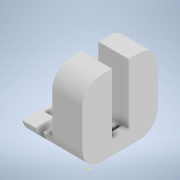
# Autodesk Inventor part: Intsragam
Saved by Autodesk Inventor 2020 (Build 240168000, 168)
## iProperties
Created: 2020-01-07
Part Number: Intsragam
Material: Générique
Document SubType Name: Modeling
Designer: laura
Density: 1 g/cm^3
Appearance: Par défaut
Author: laura
Autodesk Inventor part; units mm, degrees
ref_plane "YZ Plane" through (0, 0, 0) normal (1, 0, 0) x (0, 1, 0)
ref_plane "XZ Plane" through (0, 0, 0) normal (0, 1, 0) x (-1, 0, 0)
ref_plane "XY Plane" through (0, 0, 0) normal (0, 0, 1) x (1, 0, 0)
sketch "Esquisse1" plane through (0, 0, 0) normal (0, 1, 0) x (-1, 0, 0)
  line L0 (0, 0) -> (-40, 0)
  line L1 (-40, 0) -> (-40, -80)
  line L2 (-40, -80) -> (0, -80)
  line L3 (0, -80) -> (0, 0)
  dimension "d0" = 80
  dimension "d4" = 40
  constraints: 8 end point, 2 parallel, 1 horizontal, 1 perpendicular
  measures "d0" distance between parallel lines of L2 L0
  measures "d4" distance between parallel lines of L1 L3
extrude "Extrusion1" add sketch "Esquisse1" along normal blind 80
sketch "Esquisse2" plane through (40, 0, 0) normal (1, 0, 0) x (0, 0, -1)
  point P0 (0, 0)
sketch "Esquisse3" plane through (40, 0, 0) normal (1, 0, 0) x (0, 0, -1)
  line L0 (0, 80) -> (80, 80) projected
  line L1 (20, 20) -> (60, 20)
  line L2 (60, 20) -> (60, 80)
  line L3 (60, 80) -> (20, 80)
  line L4 (20, 80) -> (20, 20)
  line L5 (0, 0) -> (80, 0) projected
  line L6 (80, 0) -> (80, 80) projected
  line L7 (0, 0) -> (0, 80) projected
  point P0 (20, 80)
  dimension "d9" = 20
  dimension "d10" = 20
  dimension "d11" = 20
  constraints: 8 end point, 2 parallel, 1 horizontal, 1 perpendicular, 1 point on line
  measures "d9" distance between parallel lines of L5 L1
  measures "d10" distance between parallel lines of L6 L2
  measures "d11" distance between parallel lines of L7 L4
extrude "Extrusion2" cut sketch "Esquisse3" against normal blind 80 contours L0 L2 L1 L4
sketch "Esquisse4" plane through (40, 20, -20) normal (0, 1, 0) x (1, 0, 0)
  line L0 (0, 40) -> (-40, 40) projected
  line L1 (0, 0) -> (-5, 0)
  line L2 (-5, 40) -> (0, 40)
  line L3 (0, 40) -> (0, 0)
  line L4 (-5, 40) -> (-10, 40)
  line L5 (-9, 10) -> (-12, 10)
  line L6 (-12, 10) -> (-12, 30)
  line L7 (-12, 30) -> (-9, 30)
  line L8 (-9, 10) -> (-9, 30)
  point P0 (-40, -20)
  dimension "d19" = 20
  dimension "d21" = 9
  dimension "d22" = 3
  constraints: 16 end point, 2 horizontal, 2 vertical, 1 parallel, 1 point on line
  measures "d19" distance of L5.end L6.end
  measures "d21" distance between parallel lines of L8 L3
  measures "d22" distance of L5.start L5.end
extrude "Extrusion3" cut sketch "Esquisse4" against normal blind 10
sketch "Esquisse6" plane through (40, 20, -20) normal (0, 0, -1) x (-1, 0, 0)
  line L0 (40, 60) -> (40, 0) projected
  line L1 (0, 60) -> (40, 60) projected
  line L2 (0, 0) -> (0, 60) projected
  line L3 (0, 0) -> (40, 0) projected
  point P0 (40, -20)
extrude "Extrusion4" add sketch "Esquisse6" along normal blind 9
sketch "Esquisse7" plane through (40, 20, -60) normal (0, 0, 1) x (1, 0, 0)
  line L0 (-40, 0) -> (-40, 60) projected
  line L1 (0, 0) -> (-40, 0) projected
  line L2 (0, 60) -> (0, 0) projected
  line L3 (-40, 60) -> (0, 60) projected
  point P0 (-40, -20)
extrude "Extrusion5" add sketch "Esquisse7" along normal blind 9
sketch "Esquisse8" plane through (0, 80, 0) normal (0, 1, 0) x (1, 0, 0)
  line L0 (40, 51) -> (40, 80) projected
  line L1 (40, 80) -> (0, 80) projected
  line L2 (0, 80) -> (0, 51) projected
  line L3 (40, 51) -> (0, 51) projected
  point P0 (0, 0)
extrude "Extrusion6" add sketch "Esquisse8" along normal blind 20
sketch "Esquisse9" plane through (0, 80, 0) normal (0, 1, 0) x (1, 0, 0)
  line L0 (0, 29) -> (0, 0) projected
  line L1 (0, 0) -> (40, 0) projected
  line L2 (40, 0) -> (40, 29) projected
  line L3 (0, 29) -> (40, 29) projected
extrude "Extrusion7" add sketch "Esquisse9" along normal blind 20
sketch "Esquisse10" plane through (0, 0, 0) normal (0, 0, 1) x (1, 0, 0)
  line L0 (0, 0) -> (40, 0) projected
  line L1 (40, 0) -> (40, 100) projected
  line L2 (0, 100) -> (40, 100) projected
  line L3 (0, 0) -> (0, 100) projected
extrude "Extrusion8" add sketch "Esquisse10" along normal blind 10
sketch "Esquisse11" plane through (40, 0, -80) normal (0, 0, -1) x (-1, 0, 0)
  line L0 (0, 0) -> (40, 0) projected
  line L1 (40, 0) -> (40, 100) projected
  line L2 (0, 100) -> (40, 100) projected
  line L3 (0, 0) -> (0, 100) projected
extrude "Extrusion9" add sketch "Esquisse11" along normal blind 10
sketch "Esquisse12" plane through (0, 20, -51) normal (-1, 0, 0) x (0, 0, 1)
  line L0 (22, 80) -> (61, 80) projected
  line L1 (61, 80) -> (36, 80)
  line L2 (61, 80) -> (61, 55)
  line L3 (61, 80) -> (61, -20) projected
  arc A0 (61, 55) -> (36, 80) centre (36, 55) ccw
  point P0 (51, -20)
  dimension "d35" = 25
  dimension "d36" = 25
  constraints: 4 end point, 2 point on circle, 2 point on line, 1 centre point, 1 tangent
  measures "d35" distance of L0.end L1.end
  measures "d36" distance of L0.end L2.end
ref_plane "Plan de construction1" through (40, 0, -40) normal (0, 0, -1) x (-1, 0, 0)
extrude "Extrusion10" cut sketch "Esquisse12" against normal up to surface (40 mm away)
mirror "Symétrie1" about plane through (40, 0, -40) normal (0, 0, -1) of "Extrusion10"
ref_plane "Plan de construction2" through (0, 50, 0) normal (0, 1, 0) x (1, 0, 0)
mirror "Symétrie2" about plane through (0, 50, 0) normal (0, 1, 0) of "Extrusion10", "Symétrie1"
sketch "Esquisse13" plane through (0, 20, -51) normal (-1, 0, 0) x (0, 0, 1)
  line L0 (11, -10) -> (-14, -10)
  line L1 (11, -10) -> (36, -10)
  line L2 (-14, -10) -> (-14, 0)
  line L3 (-14, 0) -> (-38.4949, 0)
  line L4 (36, -10) -> (36, 0)
  line L5 (36, 0) -> (60.4949, 0)
  arc A0 (-38.4949, 0) -> (-14, -20) centre (-14, 5) ccw
  arc A1 (36, -20) -> (60.4949, 0) centre (36, 5) ccw
  line L6 (36, -20) -> (-14, -20)
  point P0 (51, -20)
  dimension "d40" = 25
  dimension "d41" = 25
  dimension "d42" = 10
  constraints: 14 end point, 4 point on circle, 2 centre point, 2 point on line
  measures "d40" distance of L0.start L0.end
  measures "d41" distance of L0.start L1.end
  measures "d42" distance of L0.end L2.end
extrude "Extrusion11" add sketch "Esquisse13" along normal blind 40
sketch "Esquisse14" plane through (0, 10, -15) normal (0, 1, 0) x (1, 0, 0)
  line L0 (-40, 0) -> (-40, 50) projected
  line L1 (40, 0) -> (-40, 0) projected
  line L2 (-40, 50) -> (-35, 50)
  line L3 (-35, 50) -> (-35, 0)
  line L4 (-35, 0) -> (-40, 0)
  line L5 (-40, 0) -> (-40, 50)
  point P0 (0, -15)
  dimension "d45" = 5
  constraints: 8 end point, 2 parallel, 1 horizontal, 1 perpendicular, 1 point on line
  measures "d45" distance of L3.end L4.end
extrude "Extrusion12" add sketch "Esquisse14" along normal up to surface (10 mm away)
sketch "Esquisse15" plane through (0, 20, 9.4949) normal (0, 1, 0) x (1, 0, 0)
  line L0 (-17.5, 24.4949) -> (-12.5, 24.4949)
  line L1 (-12.5, 24.4949) -> (-22.5, 24.4949)
  line L2 (-22.5, 24.4949) -> (-22.5, 0)
  line L3 (-12.5, 24.4949) -> (-12.5, 0)
  line L4 (-22.5, 0) -> (-12.5, 0)
  dimension "d48" = 5
  dimension "d49" = 10
  constraints: 10 end point, 2 perpendicular, 1 parallel
  measures "d48" distance of L0.start L0.end
  measures "d49" distance of L0.end L1.end
extrude "Extrusion13" cut sketch "Esquisse15" against normal up to surface (10 mm away)
sketch "Esquisse16" plane through (40, 20, -51) normal (0, 0, 1) x (1, 0, 0)
  point P0 (-40, -20)
sketch "Esquisse17" plane through (31, 20, -50) normal (-1, 0, 0) x (0, 0, 1)
  line L0 (0, 0) -> (20, 0) projected
  line L1 (0, 0) -> (0, -10) projected
  line L2 (0, -10) -> (20, -10) projected
  line L3 (20, 0) -> (20, -10) projected
  point P0 (50, -20)
extrude "Extrusion14" cut sketch "Esquisse17" against normal blind 1
